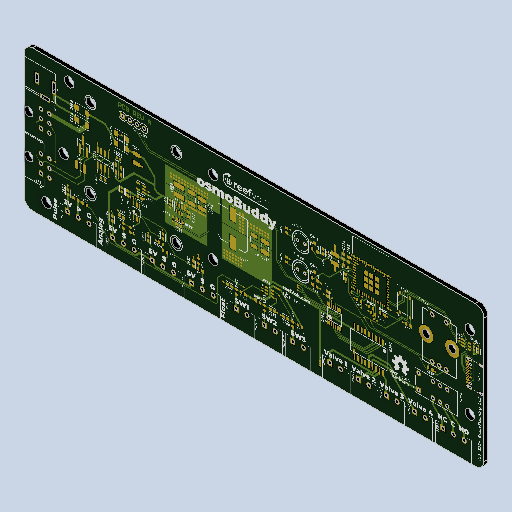
# Autodesk Inventor part: osmobuddy_v1_BOARD
Saved by Autodesk Inventor 2024.3 (Build 283343000, 343)
## iProperties
Created: 2024-08-24
Part Number: osmobuddy_v1_BOARD
Material: Generic
Document SubType Name: Modeling
Designer: atrus
Density: 1 g/cm^3
Appearance: BoardColor
Author: atrus
Autodesk Inventor part; units mm, degrees
ref_plane "YZ Plane" through (0, 0, 0) normal (1, 0, 0) x (0, 1, 0)
ref_plane "XZ Plane" through (0, 0, 0) normal (0, 1, 0) x (-1, 0, 0)
ref_plane "BoardFrontPlane" through (0, 0, 0) normal (0, 0, 1) x (1, 0, 0)
sketch "Sketch1" plane through (0, 0, 0) normal (0, 0, 1) x (1, 0, 0)
  line L0 (27, 28) -> (27, 72)
  arc A0 (30, 75) -> (27, 72) centre (30, 72) ccw
  line L1 (30, 75) -> (187, 75)
  arc A1 (190, 72) -> (187, 75) centre (187, 72) ccw
  line L2 (190, 72) -> (190, 28)
  arc A2 (187, 25) -> (190, 28) centre (187, 28) ccw
  line L3 (187, 25) -> (30, 25)
  arc A3 (27, 28) -> (30, 25) centre (30, 28) ccw
  constraints: 8 end point, 8 point on circle, 4 centre point
extrude "BoardOutline" add sketch "Sketch1" along normal blind 1.4202
sketch "img_Top" plane through (0, 0, 1.4202) normal (0, 0, 1) x (1, 0, 0)
  line L0 (27, 75) -> (190, 75) construction
  line L1 (190, 75) -> (190, 24.9849) construction
  line L2 (190, 24.9849) -> (27, 24.9849) construction
  line L3 (27, 24.9849) -> (27, 75) construction
  constraints: 2 other
decal "Decal_Top"
sketch "img_Bottom" plane through (0, 0, -1.4202) normal (0, 0, -1) x (1, 0, 0)
  line L0 (27, -25) -> (190, -25) construction
  line L1 (190, -25) -> (190, -75.0151) construction
  line L2 (190, -75.0151) -> (27, -75.0151) construction
  line L3 (27, -75.0151) -> (27, -25) construction
  constraints: 2 other
decal "Decal_Bottom"
sketch "Sketch4" plane through (0, 0, 1.4202) normal (0, 0, 1) x (1, 0, 0)
  point P0 (35.965, 57.75)
hole "J502-6" at (35.965, 57.75, 1.4202) direction (0, 0, -1) diameter 1.02 end through all
sketch "Sketch5" plane through (0, 0, 1.4202) normal (0, 0, 1) x (1, 0, 0)
  point P0 (35.965, 54.75)
hole "J502-5" at (35.965, 54.75, 1.4202) direction (0, 0, -1) diameter 1.02 end through all
sketch "Sketch6" plane through (0, 0, 1.4202) normal (0, 0, 1) x (1, 0, 0)
  point P0 (35.965, 51.75)
hole "J502-4" at (35.965, 51.75, 1.4202) direction (0, 0, -1) diameter 1.02 end through all
sketch "Sketch7" plane through (0, 0, 1.4202) normal (0, 0, 1) x (1, 0, 0)
  point P0 (32.965, 57.75)
hole "J502-3" at (32.965, 57.75, 1.4202) direction (0, 0, -1) diameter 1.02 end through all
sketch "Sketch8" plane through (0, 0, 1.4202) normal (0, 0, 1) x (1, 0, 0)
  point P0 (32.965, 54.75)
hole "J502-2" at (32.965, 54.75, 1.4202) direction (0, 0, -1) diameter 1.02 end through all
sketch "Sketch9" plane through (0, 0, 1.4202) normal (0, 0, 1) x (1, 0, 0)
  point P0 (32.965, 51.75)
hole "J502-1" at (32.965, 51.75, 1.4202) direction (0, 0, -1) diameter 1.02 end through all
sketch "Sketch10" plane through (0, 0, 1.4202) normal (0, 0, 1) x (1, 0, 0)
  point P0 (28.645, 54.75)
hole "J502-" at (28.645, 54.75, 1.4202) direction (0, 0, -1) diameter 3 end through all
sketch "Sketch11" plane through (0, 0, 1.4202) normal (0, 0, 1) x (1, 0, 0)
  point P0 (28.68, 41)
hole "J501-" at (28.68, 41, 1.4202) direction (0, 0, -1) diameter 3 end through all
sketch "Sketch12" plane through (0, 0, 1.4202) normal (0, 0, 1) x (1, 0, 0)
  point P0 (33, 38)
hole "J501-1" at (33, 38, 1.4202) direction (0, 0, -1) diameter 1.02 end through all
sketch "Sketch13" plane through (0, 0, 1.4202) normal (0, 0, 1) x (1, 0, 0)
  point P0 (33, 41)
hole "J501-2" at (33, 41, 1.4202) direction (0, 0, -1) diameter 1.02 end through all
sketch "Sketch14" plane through (0, 0, 1.4202) normal (0, 0, 1) x (1, 0, 0)
  point P0 (33, 44)
hole "J501-3" at (33, 44, 1.4202) direction (0, 0, -1) diameter 1.02 end through all
sketch "Sketch15" plane through (0, 0, 1.4202) normal (0, 0, 1) x (1, 0, 0)
  point P0 (36, 38)
hole "J501-4" at (36, 38, 1.4202) direction (0, 0, -1) diameter 1.02 end through all
sketch "Sketch16" plane through (0, 0, 1.4202) normal (0, 0, 1) x (1, 0, 0)
  point P0 (36, 41)
hole "J501-5" at (36, 41, 1.4202) direction (0, 0, -1) diameter 1.02 end through all
sketch "Sketch17" plane through (0, 0, 1.4202) normal (0, 0, 1) x (1, 0, 0)
  point P0 (36, 44)
hole "J501-6" at (36, 44, 1.4202) direction (0, 0, -1) diameter 1.02 end through all
sketch "Sketch18" plane through (0, 0, 1.4202) normal (0, 0, 1) x (1, 0, 0)
  point P0 (178.8, 57)
hole "SW400-_OCIHLIOE" at (178.8, 57, 1.4202) direction (0, 0, -1) diameter 2.6 end through all
sketch "Sketch19" plane through (0, 0, 1.4202) normal (0, 0, 1) x (1, 0, 0)
  point P0 (169.5, 57)
hole "SW400-_RHKWHGGT" at (169.5, 57, 1.4202) direction (0, 0, -1) diameter 2.6 end through all
sketch "Sketch20" plane through (0, 0, 1.4202) normal (0, 0, 1) x (1, 0, 0)
  point P0 (176.65, 64)
hole "SW400-SW2" at (176.65, 64, 1.4202) direction (0, 0, -1) diameter 1.1 end through all
sketch "Sketch21" plane through (0, 0, 1.4202) normal (0, 0, 1) x (1, 0, 0)
  point P0 (171.65, 64)
hole "SW400-SW1" at (171.65, 64, 1.4202) direction (0, 0, -1) diameter 1.1 end through all
sketch "Sketch22" plane through (0, 0, 1.4202) normal (0, 0, 1) x (1, 0, 0)
  point P0 (171.65, 49.5)
hole "SW400-A" at (171.65, 49.5, 1.4202) direction (0, 0, -1) diameter 1.1 end through all
sketch "Sketch23" plane through (0, 0, 1.4202) normal (0, 0, 1) x (1, 0, 0)
  point P0 (176.65, 49.5)
hole "SW400-B" at (176.65, 49.5, 1.4202) direction (0, 0, -1) diameter 1.1 end through all
sketch "Sketch24" plane through (0, 0, 1.4202) normal (0, 0, 1) x (1, 0, 0)
  point P0 (174.15, 49.5)
hole "SW400-C" at (174.15, 49.5, 1.4202) direction (0, 0, -1) diameter 1.1 end through all
sketch "Sketch25" plane through (0, 0, 1.4202) normal (0, 0, 1) x (1, 0, 0)
  point P0 (171.92, 43.54)
hole "K800-10" at (171.92, 43.54, 1.4202) direction (0, 0, -1) diameter 1 end through all
sketch "Sketch26" plane through (0, 0, 1.4202) normal (0, 0, 1) x (1, 0, 0)
  point P0 (174.46, 43.54)
hole "K800-9" at (174.46, 43.54, 1.4202) direction (0, 0, -1) diameter 1 end through all
sketch "Sketch27" plane through (0, 0, 1.4202) normal (0, 0, 1) x (1, 0, 0)
  point P0 (177, 43.54)
hole "K800-8" at (177, 43.54, 1.4202) direction (0, 0, -1) diameter 1 end through all
sketch "Sketch28" plane through (0, 0, 1.4202) normal (0, 0, 1) x (1, 0, 0)
  point P0 (177, 38.46)
hole "K800-5" at (177, 38.46, 1.4202) direction (0, 0, -1) diameter 1 end through all
sketch "Sketch29" plane through (0, 0, 1.4202) normal (0, 0, 1) x (1, 0, 0)
  point P0 (174.46, 38.46)
hole "K800-4" at (174.46, 38.46, 1.4202) direction (0, 0, -1) diameter 1 end through all
sketch "Sketch30" plane through (0, 0, 1.4202) normal (0, 0, 1) x (1, 0, 0)
  point P0 (171.92, 38.46)
hole "K800-3" at (171.92, 38.46, 1.4202) direction (0, 0, -1) diameter 1 end through all
sketch "Sketch31" plane through (0, 0, 1.4202) normal (0, 0, 1) x (1, 0, 0)
  point P0 (166.84, 43.54)
hole "K800-12" at (166.84, 43.54, 1.4202) direction (0, 0, -1) diameter 1 end through all
sketch "Sketch32" plane through (0, 0, 1.4202) normal (0, 0, 1) x (1, 0, 0)
  point P0 (166.84, 38.46)
hole "K800-1" at (166.84, 38.46, 1.4202) direction (0, 0, -1) diameter 1 end through all
sketch "Sketch33" plane through (0, 0, 1.4202) normal (0, 0, 1) x (1, 0, 0)
  point P0 (86.38, 31)
hole "J923-01" at (86.38, 31, 1.4202) direction (0, 0, -1) diameter 1.2 end through all
sketch "Sketch34" plane through (0, 0, 1.4202) normal (0, 0, 1) x (1, 0, 0)
  point P0 (90.19, 31)
hole "J923-02" at (90.19, 31, 1.4202) direction (0, 0, -1) diameter 1.2 end through all
sketch "Sketch35" plane through (0, 0, 1.4202) normal (0, 0, 1) x (1, 0, 0)
  point P0 (94, 31)
hole "J923-03" at (94, 31, 1.4202) direction (0, 0, -1) diameter 1.2 end through all
sketch "Sketch36" plane through (0, 0, 1.4202) normal (0, 0, 1) x (1, 0, 0)
  point P0 (175.38, 31)
hole "J804-01" at (175.38, 31, 1.4202) direction (0, 0, -1) diameter 1.2 end through all
sketch "Sketch37" plane through (0, 0, 1.4202) normal (0, 0, 1) x (1, 0, 0)
  point P0 (179.19, 31)
hole "J804-02" at (179.19, 31, 1.4202) direction (0, 0, -1) diameter 1.2 end through all
sketch "Sketch38" plane through (0, 0, 1.4202) normal (0, 0, 1) x (1, 0, 0)
  point P0 (183, 31)
hole "J804-03" at (183, 31, 1.4202) direction (0, 0, -1) diameter 1.2 end through all
sketch "Sketch39" plane through (0, 0, 1.4202) normal (0, 0, 1) x (1, 0, 0)
  point P0 (42.38, 31)
hole "J922-01" at (42.38, 31, 1.4202) direction (0, 0, -1) diameter 1.2 end through all
sketch "Sketch40" plane through (0, 0, 1.4202) normal (0, 0, 1) x (1, 0, 0)
  point P0 (46.19, 31)
hole "J922-02" at (46.19, 31, 1.4202) direction (0, 0, -1) diameter 1.2 end through all
sketch "Sketch41" plane through (0, 0, 1.4202) normal (0, 0, 1) x (1, 0, 0)
  point P0 (50, 31)
hole "J922-03" at (50, 31, 1.4202) direction (0, 0, -1) diameter 1.2 end through all
sketch "Sketch42" plane through (0, 0, 1.4202) normal (0, 0, 1) x (1, 0, 0)
  point P0 (58.38, 31)
hole "J921-01" at (58.38, 31, 1.4202) direction (0, 0, -1) diameter 1.2 end through all
sketch "Sketch43" plane through (0, 0, 1.4202) normal (0, 0, 1) x (1, 0, 0)
  point P0 (62.19, 31)
hole "J921-02" at (62.19, 31, 1.4202) direction (0, 0, -1) diameter 1.2 end through all
sketch "Sketch44" plane through (0, 0, 1.4202) normal (0, 0, 1) x (1, 0, 0)
  point P0 (66, 31)
hole "J921-03" at (66, 31, 1.4202) direction (0, 0, -1) diameter 1.2 end through all
sketch "Sketch45" plane through (0, 0, 1.4202) normal (0, 0, 1) x (1, 0, 0)
  point P0 (72.38, 31)
hole "J920-01" at (72.38, 31, 1.4202) direction (0, 0, -1) diameter 1.2 end through all
sketch "Sketch46" plane through (0, 0, 1.4202) normal (0, 0, 1) x (1, 0, 0)
  point P0 (76.19, 31)
hole "J920-02" at (76.19, 31, 1.4202) direction (0, 0, -1) diameter 1.2 end through all
sketch "Sketch47" plane through (0, 0, 1.4202) normal (0, 0, 1) x (1, 0, 0)
  point P0 (80, 31)
hole "J920-03" at (80, 31, 1.4202) direction (0, 0, -1) diameter 1.2 end through all
sketch "Sketch48" plane through (0, 0, 1.4202) normal (0, 0, 1) x (1, 0, 0)
  point P0 (165.38, 31)
hole "J803-01" at (165.38, 31, 1.4202) direction (0, 0, -1) diameter 1.2 end through all
sketch "Sketch49" plane through (0, 0, 1.4202) normal (0, 0, 1) x (1, 0, 0)
  point P0 (169.19, 31)
hole "J803-02" at (169.19, 31, 1.4202) direction (0, 0, -1) diameter 1.2 end through all
sketch "Sketch50" plane through (0, 0, 1.4202) normal (0, 0, 1) x (1, 0, 0)
  point P0 (102.19, 31)
hole "J902-01" at (102.19, 31, 1.4202) direction (0, 0, -1) diameter 1.2 end through all
sketch "Sketch51" plane through (0, 0, 1.4202) normal (0, 0, 1) x (1, 0, 0)
  point P0 (106, 31)
hole "J902-02" at (106, 31, 1.4202) direction (0, 0, -1) diameter 1.2 end through all
sketch "Sketch52" plane through (0, 0, 1.4202) normal (0, 0, 1) x (1, 0, 0)
  point P0 (112.19, 31)
hole "J901-01" at (112.19, 31, 1.4202) direction (0, 0, -1) diameter 1.2 end through all
sketch "Sketch53" plane through (0, 0, 1.4202) normal (0, 0, 1) x (1, 0, 0)
  point P0 (116, 31)
hole "J901-02" at (116, 31, 1.4202) direction (0, 0, -1) diameter 1.2 end through all
sketch "Sketch54" plane through (0, 0, 1.4202) normal (0, 0, 1) x (1, 0, 0)
  point P0 (122.19, 31)
hole "J900-01" at (122.19, 31, 1.4202) direction (0, 0, -1) diameter 1.2 end through all
sketch "Sketch55" plane through (0, 0, 1.4202) normal (0, 0, 1) x (1, 0, 0)
  point P0 (126, 31)
hole "J900-02" at (126, 31, 1.4202) direction (0, 0, -1) diameter 1.2 end through all
sketch "Sketch56" plane through (0, 0, 1.4202) normal (0, 0, 1) x (1, 0, 0)
  point P0 (135.38, 31)
hole "J802-01" at (135.38, 31, 1.4202) direction (0, 0, -1) diameter 1.2 end through all
sketch "Sketch57" plane through (0, 0, 1.4202) normal (0, 0, 1) x (1, 0, 0)
  point P0 (139.19, 31)
hole "J802-02" at (139.19, 31, 1.4202) direction (0, 0, -1) diameter 1.2 end through all
sketch "Sketch58" plane through (0, 0, 1.4202) normal (0, 0, 1) x (1, 0, 0)
  point P0 (145.38, 31)
hole "J801-01" at (145.38, 31, 1.4202) direction (0, 0, -1) diameter 1.2 end through all
sketch "Sketch59" plane through (0, 0, 1.4202) normal (0, 0, 1) x (1, 0, 0)
  point P0 (149.19, 31)
hole "J801-02" at (149.19, 31, 1.4202) direction (0, 0, -1) diameter 1.2 end through all
sketch "Sketch60" plane through (0, 0, 1.4202) normal (0, 0, 1) x (1, 0, 0)
  point P0 (155.38, 31)
hole "J800-01" at (155.38, 31, 1.4202) direction (0, 0, -1) diameter 1.2 end through all
sketch "Sketch61" plane through (0, 0, 1.4202) normal (0, 0, 1) x (1, 0, 0)
  point P0 (159.19, 31)
hole "J800-02" at (159.19, 31, 1.4202) direction (0, 0, -1) diameter 1.2 end through all
sketch "Sketch62" plane through (0, 0, 1.4202) normal (0, 0, 1) x (1, 0, 0)
  point P0 (124, 63)
hole "LED401-A" at (124, 63, 1.4202) direction (0, 0, -1) diameter 0.8128 end through all
sketch "Sketch63" plane through (0, 0, 1.4202) normal (0, 0, 1) x (1, 0, 0)
  point P0 (126.54, 63)
hole "LED401-C" at (126.54, 63, 1.4202) direction (0, 0, -1) diameter 0.8128 end through all
sketch "Sketch64" plane through (0, 0, 1.4202) normal (0, 0, 1) x (1, 0, 0)
  point P0 (124, 54)
hole "LED400-A" at (124, 54, 1.4202) direction (0, 0, -1) diameter 0.8128 end through all
sketch "Sketch65" plane through (0, 0, 1.4202) normal (0, 0, 1) x (1, 0, 0)
  point P0 (126.54, 54)
hole "LED400-C" at (126.54, 54, 1.4202) direction (0, 0, -1) diameter 0.8128 end through all
sketch "Sketch66" plane through (0, 0, 1.4202) normal (0, 0, 1) x (1, 0, 0)
  point P0 (185.286, 49.694)
hole "J700-_NIPGLSKT" at (185.286, 49.694, 1.4202) direction (0, 0, -1) diameter 0.65 end through all
sketch "Sketch67" plane through (0, 0, 1.4202) normal (0, 0, 1) x (1, 0, 0)
  point P0 (185.286, 55.474)
hole "J700-_AUUUXLFT" at (185.286, 55.474, 1.4202) direction (0, 0, -1) diameter 0.65 end through all
sketch "Sketch68" plane through (0, 0, 1.4202) normal (0, 0, 1) x (1, 0, 0)
  line L0 (189.366, 56.904) -> (188.566, 56.904) construction
  line L1 (189.366, 57.204) -> (188.566, 57.204)
  line L2 (188.566, 56.604) -> (189.366, 56.604)
  arc A0 (189.366, 56.604) -> (189.366, 57.204) centre (189.366, 56.904) ccw
  arc A1 (188.566, 57.204) -> (188.566, 56.604) centre (188.566, 56.904) ccw
  point P0 (188.966, 56.904)
  constraints: 8 end point, 4 point on circle, 4 tangent, 2 centre point, 1 midpoint, 1 parallel
extrude "J700-SH4" cut sketch "Sketch68" against normal through all
sketch "Sketch69" plane through (0, 0, 1.4202) normal (0, 0, 1) x (1, 0, 0)
  line L0 (189.366, 48.264) -> (188.566, 48.264) construction
  line L1 (189.366, 48.564) -> (188.566, 48.564)
  line L2 (188.566, 47.964) -> (189.366, 47.964)
  arc A0 (189.366, 47.964) -> (189.366, 48.564) centre (189.366, 48.264) ccw
  arc A1 (188.566, 48.564) -> (188.566, 47.964) centre (188.566, 48.264) ccw
  point P0 (188.966, 48.264)
  constraints: 8 end point, 4 point on circle, 4 tangent, 2 centre point, 1 midpoint, 1 parallel
extrude "J700-SH3" cut sketch "Sketch69" against normal through all
sketch "Sketch70" plane through (0, 0, 1.4202) normal (0, 0, 1) x (1, 0, 0)
  line L0 (185.336, 56.904) -> (184.236, 56.904) construction
  line L1 (185.336, 57.204) -> (184.236, 57.204)
  line L2 (184.236, 56.604) -> (185.336, 56.604)
  arc A0 (185.336, 56.604) -> (185.336, 57.204) centre (185.336, 56.904) ccw
  arc A1 (184.236, 57.204) -> (184.236, 56.604) centre (184.236, 56.904) ccw
  point P0 (184.786, 56.904)
  constraints: 8 end point, 4 point on circle, 4 tangent, 2 centre point, 1 midpoint, 1 parallel
extrude "J700-SH2" cut sketch "Sketch70" against normal through all
sketch "Sketch71" plane through (0, 0, 1.4202) normal (0, 0, 1) x (1, 0, 0)
  line L0 (185.336, 48.264) -> (184.236, 48.264) construction
  line L1 (185.336, 48.564) -> (184.236, 48.564)
  line L2 (184.236, 47.964) -> (185.336, 47.964)
  arc A0 (185.336, 47.964) -> (185.336, 48.564) centre (185.336, 48.264) ccw
  arc A1 (184.236, 48.564) -> (184.236, 47.964) centre (184.236, 48.264) ccw
  point P0 (184.786, 48.264)
  constraints: 8 end point, 4 point on circle, 4 tangent, 2 centre point, 1 midpoint, 1 parallel
extrude "J700-SH1" cut sketch "Sketch71" against normal through all
sketch "Sketch72" plane through (0, 0, 1.4202) normal (0, 0, 1) x (1, 0, 0)
  line L0 (37.5, 65.25) -> (37.5, 67.75) construction
  line L1 (38, 65.25) -> (38, 67.75)
  line L2 (37, 67.75) -> (37, 65.25)
  arc A0 (37, 65.25) -> (38, 65.25) centre (37.5, 65.25) ccw
  arc A1 (38, 67.75) -> (37, 67.75) centre (37.5, 67.75) ccw
  point P0 (37.5, 66.5)
  constraints: 8 end point, 4 point on circle, 4 tangent, 2 centre point, 1 midpoint, 1 parallel
extrude "J500-1" cut sketch "Sketch72" against normal through all
sketch "Sketch73" plane through (0, 0, 1.4202) normal (0, 0, 1) x (1, 0, 0)
  line L0 (31.5, 65.5) -> (31.5, 67.5) construction
  line L1 (32, 65.5) -> (32, 67.5)
  line L2 (31, 67.5) -> (31, 65.5)
  arc A0 (31, 65.5) -> (32, 65.5) centre (31.5, 65.5) ccw
  arc A1 (32, 67.5) -> (31, 67.5) centre (31.5, 67.5) ccw
  point P0 (31.5, 66.5)
  constraints: 8 end point, 4 point on circle, 4 tangent, 2 centre point, 1 midpoint, 1 parallel
extrude "J500-2" cut sketch "Sketch73" against normal through all
sketch "Sketch74" plane through (0, 0, 1.4202) normal (0, 0, 1) x (1, 0, 0)
  line L0 (35.5, 61.8) -> (33.5, 61.8) construction
  line L1 (35.5, 62.3) -> (33.5, 62.3)
  line L2 (33.5, 61.3) -> (35.5, 61.3)
  arc A0 (35.5, 61.3) -> (35.5, 62.3) centre (35.5, 61.8) ccw
  arc A1 (33.5, 62.3) -> (33.5, 61.3) centre (33.5, 61.8) ccw
  point P0 (34.5, 61.8)
  constraints: 8 end point, 4 point on circle, 4 tangent, 2 centre point, 1 midpoint, 1 parallel
extrude "J500-3" cut sketch "Sketch74" against normal through all
sketch "Sketch75" plane through (0, 0, 1.4202) normal (0, 0, 1) x (1, 0, 0)
  point P0 (50.49, 68.476)
hole "DISP200-_LQCEIGQV" at (50.49, 68.476, 1.4202) direction (0, 0, -1) diameter 3.048 end through all
sketch "Sketch76" plane through (0, 0, 1.4202) normal (0, 0, 1) x (1, 0, 0)
  point P0 (61.92, 70)
hole "DISP200-1" at (61.92, 70, 1.4202) direction (0, 0, -1) diameter 1.016 end through all
sketch "Sketch77" plane through (0, 0, 1.4202) normal (0, 0, 1) x (1, 0, 0)
  point P0 (64.46, 70)
hole "DISP200-2" at (64.46, 70, 1.4202) direction (0, 0, -1) diameter 1.016 end through all
sketch "Sketch78" plane through (0, 0, 1.4202) normal (0, 0, 1) x (1, 0, 0)
  point P0 (67, 70)
hole "DISP200-3" at (67, 70, 1.4202) direction (0, 0, -1) diameter 1.016 end through all
sketch "Sketch79" plane through (0, 0, 1.4202) normal (0, 0, 1) x (1, 0, 0)
  point P0 (69.54, 70)
hole "DISP200-4" at (69.54, 70, 1.4202) direction (0, 0, -1) diameter 1.016 end through all
sketch "Sketch80" plane through (0, 0, 1.4202) normal (0, 0, 1) x (1, 0, 0)
  point P0 (80.97, 68.476)
hole "DISP200-_LOWYJAUG" at (80.97, 68.476, 1.4202) direction (0, 0, -1) diameter 3.048 end through all
sketch "Sketch81" plane through (0, 0, 1.4202) normal (0, 0, 1) x (1, 0, 0)
  point P0 (80.97, 40.536)
hole "DISP200-_LARHPKQX" at (80.97, 40.536, 1.4202) direction (0, 0, -1) diameter 3.048 end through all
sketch "Sketch82" plane through (0, 0, 1.4202) normal (0, 0, 1) x (1, 0, 0)
  point P0 (50.49, 40.536)
hole "DISP200-_GIWYTPNR" at (50.49, 40.536, 1.4202) direction (0, 0, -1) diameter 3.048 end through all
sketch "Sketch83" plane through (0, 0, 1.4202) normal (0, 0, 1) x (1, 0, 0)
  point P0 (43, 71)
hole "Free-3_RJFAJGEP" at (43, 71, 1.4202) direction (0, 0, -1) diameter 3.4 end through all
sketch "Sketch84" plane through (0, 0, 1.4202) normal (0, 0, 1) x (1, 0, 0)
  point P0 (94, 42)
hole "Free-5" at (94, 42, 1.4202) direction (0, 0, -1) diameter 3.4 end through all
sketch "Sketch85" plane through (0, 0, 1.4202) normal (0, 0, 1) x (1, 0, 0)
  point P0 (41, 48)
hole "Free-3_RLCIVFQN" at (41, 48, 1.4202) direction (0, 0, -1) diameter 3.4 end through all
sketch "Sketch86" plane through (0, 0, 1.4202) normal (0, 0, 1) x (1, 0, 0)
  point P0 (185, 40)
hole "Free-7" at (185, 40, 1.4202) direction (0, 0, -1) diameter 3.4 end through all
sketch "Sketch87" plane through (0, 0, 1.4202) normal (0, 0, 1) x (1, 0, 0)
  point P0 (94, 68)
hole "Free-6" at (94, 68, 1.4202) direction (0, 0, -1) diameter 3.4 end through all
sketch "Sketch88" plane through (0, 0, 1.4202) normal (0, 0, 1) x (1, 0, 0)
  point P0 (185, 66)
hole "Free-4" at (185, 66, 1.4202) direction (0, 0, -1) diameter 3.4 end through all
sketch "Sketch89" plane through (0, 0, 1.4202) normal (0, 0, 1) x (1, 0, 0)
  point P0 (35, 30)
hole "Free-2" at (35, 30, 1.4202) direction (0, 0, -1) diameter 3.4 end through all
sketch "Sketch90" plane through (0, 0, 1.4202) normal (0, 0, 1) x (1, 0, 0)
  line L0 (20.25, 33) -> (106.75, 33)
  line L1 (106.75, 33) -> (106.75, 72)
  line L2 (106.75, 72) -> (20.25, 72)
  line L3 (20.25, 72) -> (20.25, 33)
  constraints: 8 end point
surface extrude "U_dcb_single_input" sketch "Sketch90" along normal blind 0.0508 shown yes curves L0 L1 L2 L3
sketch "Sketch91" plane through (0, 0, 1.4202) normal (0, 0, 1) x (1, 0, 0)
  line L0 (58.25, 45.25) -> (114.75, 45.25)
  line L1 (114.75, 45.25) -> (114.75, 65.5)
  line L2 (114.75, 65.5) -> (58.25, 65.5)
  line L3 (58.25, 65.5) -> (58.25, 45.25)
  constraints: 8 end point
surface extrude "U_dcdc_60v_12v" sketch "Sketch91" along normal blind 0.0508 shown yes curves L0 L1 L2 L3
sketch "Sketch92" plane through (0, 0, 1.4202) normal (0, 0, 1) x (1, 0, 0)
  line L0 (44.75, 42) -> (181.75, 42)
  line L1 (181.75, 42) -> (181.75, 74.75)
  line L2 (181.75, 74.75) -> (44.75, 74.75)
  line L3 (44.75, 74.75) -> (44.75, 42)
  constraints: 8 end point
surface extrude "U_dcb_lite_logic" sketch "Sketch92" along normal blind 0.0508 shown yes curves L0 L1 L2 L3
sketch "Sketch93" plane through (0, 0, 1.4202) normal (0, 0, 1) x (1, 0, 0)
  line L0 (131.5, 12.5) -> (186.25, 12.5)
  line L1 (186.25, 12.5) -> (186.25, 48.25)
  line L2 (186.25, 48.25) -> (131.5, 48.25)
  line L3 (131.5, 48.25) -> (131.5, 12.5)
  constraints: 8 end point
surface extrude "U_solenoid_channels" sketch "Sketch93" along normal blind 0.0508 shown yes curves L0 L1 L2 L3
sketch "Sketch94" plane through (0, 0, 1.4202) normal (0, 0, 1) x (1, 0, 0)
  line L0 (38.5, 12.5) -> (97.25, 12.5)
  line L1 (97.25, 12.5) -> (97.25, 42.25)
  line L2 (97.25, 42.25) -> (38.5, 42.25)
  line L3 (38.5, 42.25) -> (38.5, 12.5)
  constraints: 8 end point
surface extrude "U_pressure_input" sketch "Sketch94" along normal blind 0.0508 shown yes curves L0 L1 L2 L3
sketch "Sketch95" plane through (0, 0, 1.4202) normal (0, 0, 1) x (1, 0, 0)
  line L0 (180.75, 47) -> (192.25, 47)
  line L1 (192.25, 47) -> (192.25, 62.75)
  line L2 (192.25, 62.75) -> (180.75, 62.75)
  line L3 (180.75, 62.75) -> (180.75, 47)
  constraints: 8 end point
surface extrude "U_usb_input" sketch "Sketch95" along normal blind 0.0508 shown yes curves L0 L1 L2 L3
sketch "Sketch96" plane through (0, 0, 1.4202) normal (0, 0, 1) x (1, 0, 0)
  line L0 (97.75, 12.75) -> (129.25, 12.75)
  line L1 (129.25, 12.75) -> (129.25, 44)
  line L2 (129.25, 44) -> (97.75, 44)
  line L3 (97.75, 44) -> (97.75, 12.75)
  constraints: 8 end point
surface extrude "U_switch_input" sketch "Sketch96" along normal blind 0.0508 shown yes curves L0 L1 L2 L3
sketch "Sketch97" plane through (0, 0, 1.4202) normal (0, 0, 1) x (1, 0, 0)
  line L0 (60.5, 39) -> (69, 39)
  line L1 (69, 39) -> (69, 49.25)
  line L2 (69, 49.25) -> (60.5, 49.25)
  line L3 (60.5, 49.25) -> (60.5, 39)
  constraints: 8 end point
surface extrude "U_dcb_lite_adc" sketch "Sketch97" along normal blind 0.0508 shown yes curves L0 L1 L2 L3
sketch "Sketch98" plane through (0, 0, 1.4202) normal (0, 0, 1) x (1, 0, 0)
  line L0 (47.651, 37.67) -> (47.651, 71.778)
  line L1 (47.651, 71.778) -> (83.809, 71.778)
  line L2 (83.809, 71.778) -> (83.809, 37.67)
  line L3 (83.809, 37.67) -> (47.651, 37.67)
  constraints: 8 end point
surface extrude "U_dcb_i2c_ext" sketch "Sketch98" along normal blind 0.0508 shown yes curves L0 L1 L2 L3
body "Solid1"
body "Srf1"
body "Srf2"
body "Srf3"
body "Srf4"
body "Srf5"
body "Srf6"
body "Srf7"
body "Srf8"
body "Srf9"
